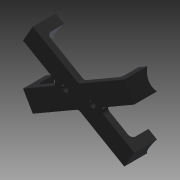
# Autodesk Inventor part: Motor Support
Saved by Autodesk Inventor 2015 (Build 190159000, 159)
## iProperties
Created: 2016-10-31
Part Number: Motor Support
Material: Generic
Document SubType Name: Modeling
Designer: James Yelland
Density: 1 g/cm^3
Appearance: Default
Author: James Yelland
Autodesk Inventor part; units mm, degrees
ref_plane "YZ Plane" through (0, 0, 0) normal (1, 0, 0) x (0, 1, 0)
ref_plane "XZ Plane" through (0, 0, 0) normal (0, 1, 0) x (-1, 0, 0)
ref_plane "XY Plane" through (0, 0, 0) normal (0, 0, 1) x (1, 0, 0)
sketch "Sketch1" plane through (0, 0, 0) normal (0, 1, 0) x (-1, 0, 0)
  arc A0 (-1, 6.3509) -> (1, 6.3509) centre (0, 8.0829) ccw
  arc A1 (-12.9998, -1.7321) -> (-12.9998, 1.7321) centre (-13.9998, 0) ccw
  arc A2 (1, -6.3509) -> (-1, -6.3509) centre (0, -8.0829) ccw
  arc A3 (13, 1.7321) -> (13, -1.7321) centre (14, 0) ccw
  circle A4 centre (7, 0) radius 1.6
  circle A5 centre (-7, 0) radius 1.6
  line L0 (0, 0) -> (26.1212, -14.7541)
  line L1 (0, 0) -> (25.9808, 15)
  line L2 (0, 0) -> (30, 0) construction
  line L3 (0, 0) -> (-25.9808, -15)
  line L4 (0, 0) -> (-25.9808, 15)
  line L5 (0, 0) -> (30, 0) construction
  line L6 (25.9808, 15) -> (28.4808, 10.6699)
  line L7 (25.9808, 15) -> (23.4808, 19.3301)
  line L8 (1, 6.3509) -> (23.4808, 19.3301)
  line L9 (28.4808, 10.6699) -> (13, 1.7321)
  line L10 (13, -1.7321) -> (28.4808, -10.6699)
  line L11 (28.4808, -10.6699) -> (23.4808, -19.3301)
  line L12 (23.4808, -19.3301) -> (1, -6.3509)
  line L13 (-1, -6.3509) -> (-23.4808, -19.3301)
  line L14 (-23.4808, -19.3301) -> (-28.4807, -10.6699)
  line L15 (-28.4807, -10.6699) -> (-12.9998, -1.7321)
  line L16 (-12.9998, 1.7321) -> (-28.4807, 10.6699)
  line L17 (-28.4807, 10.6699) -> (-23.4808, 19.3301)
  line L18 (-23.4808, 19.3301) -> (-1, 6.3509)
  dimension "d0" = 3.2
  dimension "d1" = 30
  dimension "d2" = 30
  dimension "d3" = 30
  dimension "d4" = 30
  dimension "d5" = 30
  dimension "d6" = 150
  constraints: 38 end point, 8 point on circle, 6 centre point, 3 equal radius, 3 perpendicular, 2 coincident, 2 equal length, 2 horizontal, 2 point on line
  measures "d0" diameter of A4
  measures "d1" distance of L0.start L0.end
  measures "d2" distance of L0.start L1.end
  measures "d3" angle of L2 L1
  measures "d4" distance of L0.start L3.end
  measures "d5" distance of L0.start L4.end
  measures "d6" angle of L5 L4
extrude "Extrusion1" add sketch "Sketch1" along normal blind 3
sketch "Sketch2" plane through (0, 3, 0) normal (0, 1, 0) x (1, 0, 0)
  line L0 (-23.4808, -19.3301) -> (-28.4808, -10.6699)
  line L1 (-28.4808, -10.6699) -> (-24.1506, -8.1699)
  line L2 (-24.1506, -8.1699) -> (-19.1506, -16.8301)
  line L3 (-19.1506, -16.8301) -> (-23.4808, -19.3301)
  line L4 (-28.4808, -10.6699) -> (-23.4808, -19.3301) projected
  line L5 (-23.4808, 19.3301) -> (-28.4808, 10.6699)
  line L6 (-28.4808, 10.6699) -> (-24.1506, 8.1699)
  line L7 (-24.1506, 8.1699) -> (-19.1506, 16.8301)
  line L8 (-19.1506, 16.8301) -> (-23.4808, 19.3301)
  line L9 (-1, 6.3509) -> (-23.4808, 19.3301) projected
  line L10 (28.4807, 10.6699) -> (23.4808, 19.3301)
  line L11 (23.4808, 19.3301) -> (19.1506, 16.8301)
  line L12 (19.1506, 16.8301) -> (24.1506, 8.1699)
  line L13 (24.1506, 8.1699) -> (28.4807, 10.6699)
  line L14 (28.4807, -10.6699) -> (23.4808, -19.3301)
  line L15 (23.4808, -19.3301) -> (19.1506, -16.8301)
  line L16 (19.1506, -16.8301) -> (24.1506, -8.1699)
  line L17 (24.1506, -8.1699) -> (28.4807, -10.6699)
  line L18 (23.4808, -19.3301) -> (28.4807, -10.6699) projected
  point P0 (0, 0)
  dimension "d9" = 5
  dimension "d10" = 5
  dimension "d11" = 5
  dimension "d12" = 5
  constraints: 32 end point, 9 parallel, 5 perpendicular, 2 collinear
  measures "d9" distance of L0.end L1.end
  measures "d10" distance of L6.end L5.end
  measures "d11" distance of L11.end L10.end
  measures "d12" distance of L14.end L15.end
extrude "Extrusion2" add sketch "Sketch2" along normal blind 15
fillet "Fillet1" radius 2 4 edges at (-21.6506, 3, 12.5) (-21.6506, 3, -12.5) (21.6506, 3, -12.5) (21.6506, 3, 12.5)
sketch "Sketch3" plane through (-19.1506, 5, -16.8301) normal (0.8660254, 0, 0.5) x (0.5, 0, -0.8660254)
  line L0 (-10, 13) -> (0, 13) projected
  circle A0 centre (-5, 13) radius 8
  point P0 (-5, -5)
  dimension "d16" = 16
  constraints: 1 centre point, 1 midpoint
  measures "d16" diameter of A0
extrude "Extrusion3" cut sketch "Sketch3" against normal blind 13
sketch "Sketch4" plane through (23.4808, 0, -19.3301) normal (0.8660254, 0, -0.5) x (-0.5, 0, -0.8660254)
  line L0 (0, 18) -> (-9.9999, 18) projected
  circle A0 centre (-5, 18) radius 8
  point P0 (-5, 0)
  dimension "d19" = 16
  constraints: 1 centre point, 1 midpoint
  measures "d19" diameter of A0
extrude "Extrusion4" cut sketch "Sketch4" against normal blind 13
sketch "Sketch5" plane through (28.4807, 0, 10.6699) normal (0.8660254, 0, 0.5) x (0.5, 0, -0.8660254)
  line L0 (-9.9999, 18) -> (0, 18) projected
  circle A0 centre (-5, 18) radius 8
  point P0 (-4.9999, 0)
  dimension "d22" = 16
  constraints: 1 centre point, 1 midpoint
  measures "d22" diameter of A0
extrude "Extrusion5" cut sketch "Sketch5" against normal blind 10
sketch "Sketch6" plane through (-23.4808, 0, 19.3301) normal (-0.8660254, 0, 0.5) x (0.5, 0, 0.8660254)
  line L0 (0, 18) -> (-10, 18) projected
  circle A0 centre (-5, 18) radius 8
  point P0 (-5, 0)
  dimension "d25" = 16
  constraints: 1 centre point, 1 midpoint
  measures "d25" diameter of A0
extrude "Extrusion6" cut sketch "Sketch6" against normal blind 10
body "Solid1"
